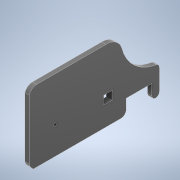
# Autodesk Inventor part: right_panel
Saved by Autodesk Inventor 2022 (Build 260153000, 153)
## iProperties
Created: 2021-06-17
Part Number: right_panel
Material: Plastic, Opaque Black
Document SubType Name: Modeling
Designer: kevin
Density: 0.952 g/cm^3
Appearance: Smooth - Black
Author: kevin
Autodesk Inventor part; units mm, degrees
ref_plane "YZ Plane" through (0, 0, 0) normal (1, 0, 0) x (0, 1, 0)
ref_plane "XZ Plane" through (0, 0, 0) normal (0, 1, 0) x (-1, 0, 0)
ref_plane "XY Plane" through (0, 0, 0) normal (0, 0, 1) x (1, 0, 0)
sketch "outline" plane through (0, 0, 0) normal (1, 0, 0) x (0, 1, 0)
  line L0 (0, 88.9038) -> (127, 88.9038) construction
  line L1 (127, 88.9038) -> (127, -88.8962) construction
  line L2 (127, -88.8962) -> (0, -88.8962) construction
  line L3 (0, -88.8962) -> (0, 88.9038) construction
  line L4 (0, 88.9038) -> (127, -88.8962) construction
  line L5 (127, 88.9038) -> (0, -88.8962) construction
  line L6 (-6.35, -82.5462) -> (38.1, -82.5462)
  line L7 (38.1, -82.5462) -> (38.1, -44.4462)
  line L8 (38.1, -44.4462) -> (-6.35, -44.4462)
  line L9 (-6.35, -44.4462) -> (-6.35, -82.5462)
  line L10 (4.9871, -50.7075) -> (22.0805, -50.7075) construction
  line L11 (22.0805, -50.7075) -> (22.0805, -80.6209) construction
  line L12 (22.0805, -80.6209) -> (4.9871, -80.6209) construction
  line L13 (4.9871, -80.6209) -> (4.9871, -50.7075) construction
  line L14 (179.262, 0.0038) -> (-38.2255, 0.0038) construction
  line L15 (0, 150.8125) -> (0, -173.0375) construction
  point P0 (63.5, 0.0038)
  point P1 (63.5, 0.0038)
  dimension "d0" = 177.8
  dimension "d1" = 127
  dimension "d2" = 38.1
  dimension "d3" = 44.45
  dimension "d4" = 6.35
  dimension "d5" = 6.35
  constraints: 24 end point, 4 horizontal, 4 parallel, 3 midpoint, 2 perpendicular, 2 vertical, 1 collinear, 1 point on line, 2 other
  measures "d0" distance of L0.end L1.end
  measures "d1" distance of L1.end L2.end
  measures "d2" distance of L8.end L6.start
  measures "d3" distance of L6.start L6.end
  measures "d4" distance between parallel lines of L6 L2
  measures "d5" distance between parallel lines of L9 L15
sketch "Sketch2" plane through (0, 0, 0) normal (1, 0, 0) x (0, 1, 0)
  line L0 (16.1492, -36.7509) -> (16.1492, 92.075)
  line L1 (25.5684, 98.5943) -> (113.7408, 98.5943)
  line L2 (121.8722, 87.4339) -> (121.8722, -14.7243)
  line L3 (38.1007, -44.45) -> (38.1007, -82.55)
  line L4 (38.1007, -44.45) -> (12.7007, -44.45)
  line L5 (38.1007, -82.55) -> (17.4632, -82.55)
  arc A0 (121.8722, 87.4339) -> (113.7408, 98.5943) centre (110.1475, 87.4339) ccw
  line L6 (31.7507, -44.45) -> (31.7507, 88.9) construction
  line L7 (25.4007, -44.45) -> (25.4007, 88.9) construction
  circle A1 centre (56.4395, 60.4012) radius 2.3813
  line L8 (0, -88.9) -> (117.475, -88.9) construction
  arc A2 (22.225, -82.55) -> (22.225, -93.6625) centre (22.225, -88.1063) ccw
  line L9 (22.225, -93.6625) -> (52.3875, -93.6625)
  arc A3 (104.2778, -38.5424) -> (58.7375, -88.9) centre (120.3654, -98.8617) ccw
  arc A4 (104.2778, -38.5424) -> (121.8722, -14.7243) centre (98.1639, -15.6185) ccw
  arc A5 (16.1492, -36.7509) -> (25.4007, -44.45) centre (23.7736, -36.9971) ccw
  arc A6 (25.5684, 98.5943) -> (16.1492, 92.075) centre (28.7116, 83.9887) ccw
  arc A7 (52.3875, -93.6625) -> (58.7375, -88.9) centre (53.0922, -87.9875) ccw
  point P0 (0, 0)
  point P1 (22.1466, -44.45)
  dimension "d6" = 6.35
  dimension "d7" = 6.35
  dimension "d8" = 4.7625
  dimension "d9" = 24.6888
  dimension "d10" = 149.3012
  constraints: 20 end point, 14 point on circle, 8 centre point, 8 horizontal, 6 vertical, 4 tangent, 2 midpoint, 2 point on line
  measures "d6" distance between parallel lines of L6 L3
  measures "d7" distance between parallel lines of L7 L6
  measures "d8" diameter of A1
  measures "d9" distance from line of L6 A1.centre
  measures "d10" distance from line of A1.centre L8
extrude "main right panel" add sketch "Sketch2" along normal blind 6.35 contours L0 A6 L1 A0 L2 A4 A3 A7 L9 A2 L5 L3 L4 A5
sketch "rat icon raw" plane through (6.35, 0, 0) normal (1, 0, 0) x (0, 0, -1)
  line L0 (-53.1267, 106.3625) -> (-10.9673, 106.3625) construction
  line L1 (-10.9673, 106.3625) -> (-10.9673, 68.2625) construction
  line L2 (-10.9673, 68.2625) -> (-53.1267, 68.2625) construction
  line L3 (-53.1267, 68.2625) -> (-53.1267, 106.3625) construction
  line L4 (-80.9625, 106.3625) -> (-14.2875, 106.3625) construction
  line L5 (-80.9625, 68.2625) -> (-14.2875, 68.2625) construction
  point P0 (0, 0)
  constraints: 4 end point, 4 horizontal, 2 collinear, 2 other
sketch "Sketch6" plane through (6.35, 0, 0) normal (1, 0, 0) x (0, 0, -1)
  line L0 (-90.482, 107.6466) -> (-76.2, 109.283)
  line L1 (-76.2, 109.283) -> (-77.7875, 104.5205)
  line L2 (-77.7875, 104.5205) -> (-82.9028, 104.5205)
  line L3 (-82.9028, 104.5205) -> (-81.9686, 96.3676)
  line L4 (-81.9686, 96.3676) -> (-86.8566, 96.3676)
  line L5 (-86.8566, 96.3676) -> (-85.1932, 104.5205)
  line L6 (-85.1932, 104.5205) -> (-91.0958, 104.5205)
  line L7 (-91.0958, 104.5205) -> (-90.482, 107.6466)
  line L8 (-73.7939, 108.2258) -> (-76.2, 96.3676)
  line L9 (-76.2, 96.3676) -> (-73.7454, 96.3676)
  line L10 (-73.7454, 96.3676) -> (-73.0058, 100.0125)
  line L11 (-73.0058, 100.0125) -> (-71.4375, 99.6943)
  line L12 (-71.4375, 99.6943) -> (-71.4375, 96.3676)
  line L13 (-71.4375, 96.3676) -> (-69.85, 96.3676)
  line L14 (-69.85, 96.3676) -> (-69.85, 101.3768)
  line L15 (-69.85, 101.3768) -> (-72.5181, 102.4162)
  line L16 (-72.5181, 102.4162) -> (-72.5181, 108.2258)
  line L17 (-72.5181, 108.2258) -> (-73.7939, 108.2258)
  line L18 (-65.1277, 100.0518) -> (-60.3603, 100.4265)
  line L19 (-60.3603, 100.4265) -> (-61.915, 103.1887)
  line L20 (-61.915, 103.1887) -> (-65.8535, 103.1887)
  line L21 (-65.8535, 103.1887) -> (-67.3493, 100.0125)
  line L22 (-67.3493, 100.0125) -> (-65.851, 96.3676)
  line L23 (-65.851, 96.3676) -> (-61.9125, 96.3676)
  line L24 (-61.9125, 96.3676) -> (-61.0199, 98.263)
  line L25 (-61.0199, 98.263) -> (-64.9627, 97.9531)
  line L26 (-64.9627, 97.9531) -> (-65.1277, 100.0518)
  line L27 (-92.0732, 92.0678) -> (-88.8982, 71.4303)
  line L28 (-88.8982, 71.4303) -> (-84.5851, 71.4303)
  line L29 (-84.5851, 71.4303) -> (-88.1511, 81.4759)
  line L30 (-88.1511, 81.4759) -> (-79.1594, 71.8603)
  line L31 (-79.1594, 71.8603) -> (-76.0148, 73.6303)
  line L32 (-76.0148, 73.6303) -> (-85.6976, 83.1021)
  line L33 (-85.6976, 83.1021) -> (-79.375, 84.8156)
  line L34 (-79.375, 84.8156) -> (-80.2421, 90.4519)
  line L35 (-80.2421, 90.4519) -> (-86.7416, 93.5127)
  line L36 (-86.7416, 93.5127) -> (-92.0732, 92.0678)
  line L37 (-88.9716, 89.5226) -> (-87.785, 85.1441)
  line L38 (-87.785, 85.1441) -> (-83.4928, 86.9084)
  line L39 (-83.4928, 86.9084) -> (-85.2835, 90.09)
  line L40 (-85.2835, 90.09) -> (-88.9716, 89.5226)
  line L41 (-64.6954, 101.9367) -> (-64.9301, 100.9638)
  line L42 (-64.9301, 100.9638) -> (-62.5497, 101.2457)
  line L43 (-62.5497, 101.2457) -> (-63.5298, 102.4036)
  line L44 (-63.5298, 102.4036) -> (-64.6954, 101.9367)
  line L45 (-76.7521, 84.3599) -> (-74.2642, 86.4657)
  line L46 (-74.2642, 86.4657) -> (-67.2415, 87.5488)
  line L47 (-67.2415, 87.5488) -> (-63.3352, 73.4152)
  line L48 (-63.3352, 73.4152) -> (-66.1281, 72.9844)
  line L49 (-66.1281, 72.9844) -> (-66.4584, 75.1263)
  line L50 (-66.4584, 75.1263) -> (-68.2934, 73.264)
  line L51 (-68.2934, 73.264) -> (-73.1451, 72.5157)
  line L52 (-73.1451, 72.5157) -> (-74.9114, 74.256)
  line L53 (-74.9114, 74.256) -> (-75.6403, 78.9817)
  line L54 (-75.6403, 78.9817) -> (-74.0283, 80.6177)
  line L55 (-74.0283, 80.6177) -> (-67.6783, 81.5971)
  line L56 (-67.6783, 81.5971) -> (-69.2347, 85.4828)
  line L57 (-69.2347, 85.4828) -> (-73.6131, 84.2727)
  line L58 (-73.6131, 84.2727) -> (-74.9869, 83.1098)
  line L59 (-74.9869, 83.1098) -> (-76.7521, 84.3599)
  line L60 (-72.0695, 78.6877) -> (-72.3134, 78.5673)
  line L61 (-72.3134, 78.5673) -> (-72.3134, 75.1263)
  line L62 (-72.3134, 75.1263) -> (-68.8702, 75.1263)
  line L63 (-68.8702, 75.1263) -> (-67.1347, 76.6189)
  line L64 (-67.1347, 76.6189) -> (-68.5083, 79.4017)
  line L65 (-68.5083, 79.4017) -> (-72.0695, 78.6877)
  line L66 (-61.8214, 93.0066) -> (-61.1645, 86.6956)
  line L67 (-61.1645, 86.6956) -> (-63.0921, 86.495)
  line L68 (-63.0921, 86.495) -> (-63.0921, 83.125)
  line L69 (-63.0921, 83.125) -> (-60.7929, 83.125)
  line L70 (-60.7929, 83.125) -> (-60.1157, 76.6189)
  line L71 (-60.1157, 76.6189) -> (-57.8831, 74.256)
  line L72 (-57.8831, 74.256) -> (-52.8496, 74.78)
  line L73 (-52.8496, 74.78) -> (-53.882, 75.8726)
  line L74 (-53.882, 75.8726) -> (-57.8951, 76.85)
  line L75 (-57.8951, 76.85) -> (-58.5482, 83.125)
  line L76 (-58.5482, 83.125) -> (-55.3914, 82.3562)
  line L77 (-55.3914, 82.3562) -> (-56.9753, 85.3316)
  line L78 (-56.9753, 85.3316) -> (-58.9439, 86.9267)
  line L79 (-59.6008, 93.2377) -> (-61.8214, 93.0066)
  line L80 (-59.6008, 93.2377) -> (-58.9439, 86.9267)
  line L81 (-90.3273, 66.9011) -> (-92.3025, 43.7452)
  line L82 (-92.3025, 43.7452) -> (-83.6552, 43.0076)
  line L83 (-83.6552, 43.0076) -> (-80.3451, 45.7207)
  line L84 (-80.3451, 45.7207) -> (-80.3451, 53.0314)
  line L85 (-80.3451, 53.0314) -> (-82.9028, 54.9333)
  line L86 (-82.9028, 54.9333) -> (-87.9789, 56.2066)
  line L87 (-87.9789, 56.2066) -> (-85.4408, 67.3056)
  line L88 (-85.4408, 67.3056) -> (-90.3273, 66.9011)
  line L89 (-89.0531, 51.5088) -> (-89.0531, 47.7554)
  line L90 (-89.0531, 47.7554) -> (-85.6389, 46.9746)
  line L91 (-85.6389, 46.9746) -> (-83.6628, 49.6321)
  line L92 (-83.6628, 49.6321) -> (-84.778, 53.0314)
  line L93 (-84.778, 53.0314) -> (-89.0531, 51.6289)
  line L94 (-77.7875, 66.9369) -> (-80.6353, 64.5461)
  line L95 (-80.6353, 64.5461) -> (-79.5703, 56.8049)
  line L96 (-79.5703, 56.8049) -> (-75.7895, 55.9249)
  line L97 (-75.7895, 55.9249) -> (-71.5386, 59.4937)
  line L98 (-71.5386, 59.4937) -> (-72.3897, 65.6805)
  line L99 (-72.3897, 65.6805) -> (-77.7875, 66.9369)
  line L100 (-77.7875, 62.5871) -> (-77.7875, 58.634)
  line L101 (-77.7875, 58.634) -> (-75.0886, 58.634)
  line L102 (-75.0886, 58.634) -> (-74.7055, 63.4204)
  line L103 (-74.7055, 63.4204) -> (-76.6131, 63.573)
  line L104 (-76.6131, 63.573) -> (-77.7875, 62.5871)
  line L105 (-68.4972, 70.5753) -> (-68.5693, 68.2366)
  line L106 (-68.5693, 68.2366) -> (-66.2151, 58.3858)
  line L107 (-66.2151, 58.3858) -> (-72.6469, 52.0948)
  line L108 (-72.6469, 52.0948) -> (-70.8707, 49.9791)
  line L109 (-70.8707, 49.9791) -> (-54.5671, 67.2736)
  line L110 (-54.5671, 67.2736) -> (-57.5505, 65.6195)
  line L111 (-57.5505, 65.6195) -> (-64.4697, 61.7832)
  line L112 (-64.4697, 61.7832) -> (-66.675, 71.0108)
  line L113 (-66.675, 71.0108) -> (-68.4972, 70.5753)
  line L114 (-43.6156, 68.0273) -> (-44.641, 70.5217)
  line L115 (-44.641, 70.5217) -> (-52.7086, 70.5217)
  line L116 (-52.7086, 70.5217) -> (-52.7086, 65.9787)
  line L117 (-52.7086, 65.9787) -> (-47.0988, 58.9781)
  line L118 (-47.0988, 58.9781) -> (-52.7086, 57.21)
  line L119 (-52.7086, 57.21) -> (-52.0224, 55.0327)
  line L120 (-52.0224, 55.0327) -> (-43.2547, 56.1214)
  line L121 (-43.2547, 56.1214) -> (-43.2547, 60.8776)
  line L122 (-43.2547, 60.8776) -> (-48.8355, 67.3792)
  line L123 (-48.8355, 67.3792) -> (-43.6156, 68.0273)
  point P0 (0, 0)
  constraints: 248 end point, 33 perpendicular, 23 parallel, 17 point on line, 6 vertical, 4 horizontal
extrude "the rat boys words" [suppressed]
sketch "detail lines" plane through (6.35, 0, 0) normal (1, 0, 0) x (0, 0, -1)
  line L0 (41.275, 68.2625) -> (-1.5875, 68.2625)
  line L1 (-1.5875, 68.2625) -> (-1.5875, 107.95)
  arc A0 (41.275, 68.2625) -> (-1.5875, 107.95) centre (-4.3356, 61.9925) ccw
  line L2 (-4.1415, 110.938) -> (-4.1415, 28.575)
  line L3 (-4.1415, 28.575) -> (31.75, 28.575)
  arc A1 (44.45, 66.675) -> (-4.1415, 110.938) centre (-10.0865, 55.6085) ccw
  line L4 (44.45, 66.675) -> (44.45, 41.275)
  arc A2 (44.45, 41.275) -> (31.75, 28.575) centre (44.45, 28.575) ccw
  line L5 (-1.5875, 61.9925) -> (4.7625, 61.9925) construction
  line L6 (-1.5875, 60.4851) -> (4.7625, 60.4851)
  line L7 (4.7625, 63.5) -> (-1.5875, 63.5)
  arc A3 (-1.5875, 63.5) -> (-1.5875, 60.4851) centre (-1.5875, 61.9925) ccw
  arc A4 (4.7625, 60.4851) -> (4.7625, 63.5) centre (4.7625, 61.9925) ccw
  line L8 (35.4697, 23.6503) -> (-87.3125, 23.6503)
  line L9 (-87.4339, 115.8875) -> (19.8438, 115.8875)
  arc A5 (33.3375, 107.95) -> (19.8438, 115.8875) centre (17.1097, 95.8012) ccw
  line L10 (-87.4339, 115.8875) -> (-87.4339, 114.3)
  line L11 (-87.4339, 114.3) -> (18.8487, 114.3)
  arc A6 (31.75, 107.1391) -> (18.8487, 114.3) centre (18.8487, 99.0979) ccw
  line L12 (31.75, 107.1391) -> (33.3375, 107.95)
  line L13 (-87.3125, 23.6503) -> (-87.3125, 21.5255)
  line L14 (-87.3125, 21.5255) -> (35.4697, 21.5255)
  line L15 (35.4697, 21.5255) -> (35.4697, 23.6503)
  point P0 (0, 0)
  point P1 (1.5875, 61.9925)
  constraints: 34 end point, 14 point on circle, 7 centre point, 5 perpendicular, 5 tangent, 4 horizontal, 4 vertical, 1 midpoint, 1 parallel
extrude "car details extrusion" add sketch "detail lines" along normal blind 2.54
sketch "rat sketch" plane through (6.35, 0, 0) normal (1, 0, 0) x (0, 0, -1)
  spline S0 degree 4 poles (-25.1113, 40.168) (-30.3286, 62.8002) (-40.2895, 47.0939) (-91.8199, 45.4722) (-69.0311, 66.7314) knots 0 0 0 0 0 1 1 1 1 1
  spline S1 degree 4 poles (-25.1113, 40.168) (-44.8827, 65.0652) (-62.3129, 21.5895) (-100.0449, 58.8688) (-70.6074, 74.0707) knots 0 0 0 0 0 1 1 1 1 1
  arc A0 (-69.0311, 66.7314) -> (-67.585, 61.8172) centre (-67.0769, 64.6366) ccw
  arc A1 (-49.2116, 58.7947) -> (-67.585, 61.8172) centre (-65.5506, 16.8269) ccw
  line L0 (-49.2116, 58.7947) -> (-50.6913, 60.6928)
  line L1 (-50.6913, 60.6928) -> (-46.1556, 58.7947)
  line L2 (-46.1556, 58.7947) -> (-48.7906, 62.1746)
  line L3 (-48.7906, 62.1746) -> (-44.7522, 60.4847)
  line L4 (-44.7522, 60.4847) -> (-47.0983, 63.4939)
  arc A2 (-55.3235, 64.9029) -> (-47.0983, 63.4939) centre (-49.5283, 74.0213) ccw
  arc A3 (-55.3235, 64.9029) -> (-61.4396, 83.2385) centre (-66.0407, 71.5159) ccw
  arc A4 (-55.3235, 64.9029) -> (-61.4396, 83.2385) centre (-62.9686, 72.5406) ccw
  arc A5 (-54.0945, 66.3736) -> (-40.9879, 66.7314) centre (-47.8743, 78.7553) ccw
  arc A6 (-40.9879, 66.7314) -> (-36.1311, 63.3712) centre (-37.5728, 66.4775) ccw
  arc A7 (-33.4791, 95.4623) -> (-76.7213, 69.5945) centre (-48.4257, 71.3709) ccw
  arc A8 (-36.1311, 63.3712) -> (-34.9888, 58.791) centre (16.1312, 73.9736) ccw
  line L5 (-34.9888, 58.791) -> (-34.9888, 62.1708)
  line L6 (-34.9888, 62.1708) -> (-32.1742, 61.0684)
  line L7 (-32.1742, 61.0684) -> (-30.8802, 58.791)
  line L8 (-30.8802, 58.791) -> (-31.2041, 61.6196)
  line L9 (-31.2041, 61.6196) -> (-32.1742, 62.8915)
  line L10 (-32.1742, 62.8915) -> (-30.6857, 62.8915)
  line L11 (-30.6857, 62.8915) -> (-29.0402, 60.4346)
  line L12 (-29.0402, 60.4346) -> (-29.0402, 62.3815)
  line L13 (-29.0402, 62.3815) -> (-29.9306, 63.7109)
  line L14 (-29.9306, 63.7109) -> (-27.2529, 62.8915)
  line L15 (-27.2529, 62.8915) -> (-28.2579, 64.392)
  arc A9 (-28.2579, 64.392) -> (-33.7777, 64.8449) centre (-31.6378, 57.0631) ccw
  arc A10 (-34.8841, 70.1283) -> (-33.7777, 64.8449) centre (-32.3651, 67.8983) ccw
  arc A11 (-34.8841, 70.1283) -> (-23.8004, 78.7218) centre (-46.3737, 96.3917) ccw
  arc A12 (-23.8004, 78.7218) -> (-15.5306, 77.1344) centre (-17.1285, 91.1448) ccw
  line L16 (-15.5306, 77.1344) -> (-13.4262, 78.7736)
  arc A13 (-13.4262, 78.7736) -> (-12.5498, 83.2524) centre (-12.73, 80.9625) ccw
  line L17 (-12.5498, 83.2524) -> (-17.1338, 91.6691)
  line L18 (-17.1338, 91.6691) -> (-22.5552, 93.9422)
  arc A14 (-24.7828, 98.5157) -> (-22.5552, 93.9422) centre (-22.0776, 97.0041) ccw
  arc A15 (-24.7828, 98.5157) -> (-27.2583, 102.3227) centre (-27.0229, 99.7674) ccw
  arc A16 (-30.6895, 96.6707) -> (-27.2583, 102.3227) centre (-32.5957, 101.6955) ccw
  arc A17 (-30.6895, 96.6707) -> (-33.4791, 95.4623) centre (-19.0133, 65.8926) ccw
  arc A18 (-17.8515, 86.2944) -> (-24.7683, 89.3504) centre (-22.6941, 84.6895) ccw
  arc A19 (-24.7558, 89.356) -> (-17.8515, 86.2944) centre (-19.1737, 92.6286) ccw
  arc A20 (-32.5957, 93.9422) -> (-29.4854, 87.2366) centre (-28.196, 91.9088) ccw
  arc A21 (-25.7638, 91.6691) -> (-32.5957, 93.9422) centre (-30.7455, 88.0996) ccw
  arc A22 (-26.408, 91.1448) -> (-31.0346, 92.4063) centre (-29.6597, 88.3339) ccw
  arc A23 (-31.0346, 92.4063) -> (-29.0402, 87.4607) centre (-25.1113, 91.9201) ccw
  line L19 (-29.0402, 87.4607) -> (-29.4854, 87.2366)
  line L20 (-26.408, 91.1448) -> (-25.7638, 91.6691)
  line L21 (-19.1737, 77.1927) -> (-22.6941, 72.5406)
  line L22 (-22.6941, 72.5406) -> (-22.6941, 71.6578)
  line L23 (-22.6941, 71.6578) -> (-18.6565, 77.1266)
  line L24 (-20.5712, 69.8924) -> (-17.5596, 76.9468)
  line L25 (-20.5712, 69.8924) -> (-20.5712, 70.2775)
  line L26 (-20.5712, 70.2775) -> (-17.8411, 77.0616)
  line L27 (-17.5935, 76.8675) -> (-18.3698, 71.0148)
  line L28 (-18.3698, 71.0148) -> (-18.1898, 70.2775)
  line L29 (-18.1898, 70.2775) -> (-17.2434, 76.8211)
  line L30 (-17.2434, 76.8211) -> (-17.2434, 77.0441)
  line L31 (-12.5498, 83.2524) -> (-9.4887, 86.2944)
  line L32 (-9.4887, 86.2944) -> (-11.9194, 84.6895)
  line L33 (-11.9194, 84.6895) -> (-6.9637, 91.1448)
  line L34 (-6.9637, 91.1448) -> (-12.5498, 85.492)
  line L35 (-12.5498, 85.492) -> (-11.3289, 88.6625)
  line L36 (-11.3289, 88.6625) -> (-13.0786, 85.5794)
  line L37 (-13.0786, 85.5794) -> (-13.5578, 85.1032)
  point P0 (0, 0)
  point P1 (-32.5957, 51.1893)
  point P2 (-50.6956, 51.4518)
  point P3 (-71.9355, 54.0894)
  point P4 (-46.3737, 47.5886)
  point P5 (-67.5516, 46.5674)
  point P6 (-79.7754, 55.7354)
  point P7 (-18.6565, 77.1266)
  constraints: 76 end point, 56 point on circle, 24 centre point, 6 parallel, 5 vertical, 3 point on line, 2 tangent, 1 coincident, 1 horizontal, 1 perpendicular, 14 other
extrude "rat extrusion" [suppressed]
mirror "Mirror1" about plane through (0, 0, 0) normal (1, 0, 0) remove original yes
sketch "Sketch7" plane through (-6.35, 25.5684, 98.5943) normal (-1, 0, 0) x (0, 0, 1)
  line L0 (-83.8164, 82.6102) -> (-17.4625, 82.6102) construction
  line L1 (-17.4625, 82.6102) -> (-17.4625, 36.5125) construction
  line L2 (-17.4625, 36.5125) -> (-83.8164, 36.5125) construction
  line L3 (-83.8164, 36.5125) -> (-83.8164, 82.6102) construction
  line L4 (-82.8534, 82.6102) -> (-79.4482, 82.6102)
  spline S0 degree 2 poles (-79.4482, 82.6102) (-76.043, 82.6102) (-73.6287, 82.0799) (-72.1075, 79.9168) (-72.1075, 77.5583) knots 0 0 0 1 2 3 3 3
  spline S1 degree 2 poles (-72.1075, 77.5583) (-72.1075, 75.3951) (-73.1821, 73.9018) (-74.7591, 73.7483) knots 0 0 0 1 2 2 2
  spline S2 degree 2 poles (-74.7591, 73.7483) (-73.3356, 73.3994) (-72.3447, 72.2132) (-72.1075, 71.2223) (-72.1075, 68.9755) knots 0 0 0 1 2 3 3 3
  line L5 (-72.1075, 68.9755) -> (-72.1075, 64.0909)
  line L6 (-72.1075, 64.0909) -> (-76.5873, 64.0909)
  line L7 (-76.5873, 64.0909) -> (-76.5873, 70.2454)
  spline S3 degree 2 poles (-76.5873, 70.2454) (-76.5873, 71.7247) (-77.0478, 72.4365) (-78.0387, 72.4365) knots 0 0 0 1 2 2 2
  line L8 (-78.0387, 72.4365) -> (-78.0387, 64.0909)
  line L9 (-78.0387, 64.0909) -> (-82.8534, 64.0909)
  line L10 (-82.8534, 64.0909) -> (-82.8534, 82.6102)
  line L11 (-78.0387, 79.4423) -> (-78.0387, 75.3253)
  spline S4 degree 2 poles (-78.0387, 75.3253) (-77.2293, 75.3253) (-76.5873, 75.7719) (-76.5873, 77) knots 0 0 0 1 2 2 2
  line L12 (-76.5873, 77) -> (-76.5873, 78.0188)
  spline S5 degree 2 poles (-76.5873, 78.0188) (-76.5873, 78.898) (-77.2153, 79.4423) (-78.0387, 79.4423) knots 0 0 0 1 2 2 2
  line L13 (-61.9198, 82.6102) -> (-59.1565, 64.0909)
  line L14 (-59.1565, 64.0909) -> (-64.0969, 64.0909)
  line L15 (-64.0969, 64.0909) -> (-64.3481, 67.4264)
  line L16 (-64.3481, 67.4264) -> (-66.0646, 67.4264)
  line L17 (-66.0646, 67.4264) -> (-66.3438, 64.0909)
  line L18 (-66.3438, 64.0909) -> (-71.3399, 64.0909)
  line L19 (-71.3399, 64.0909) -> (-68.8977, 82.6102)
  line L20 (-68.8977, 82.6102) -> (-61.9198, 82.6102)
  spline S6 degree 2 poles (-64.4737, 70.706) (-64.8226, 73.846) (-65.1994, 78.4793) knots 0 0 0 1 1 1
  spline S7 degree 2 poles (-65.1994, 78.4793) (-65.9251, 73.1622) (-66.1205, 70.706) knots 0 0 0 1 1 1
  line L21 (-66.1205, 70.706) -> (-64.4737, 70.706)
  line L22 (-48.6339, 82.6102) -> (-48.6339, 78.898)
  line L23 (-48.6339, 78.898) -> (-51.4948, 78.898)
  line L24 (-51.4948, 78.898) -> (-51.4948, 64.0909)
  line L25 (-51.4948, 64.0909) -> (-56.3096, 64.0909)
  line L26 (-56.3096, 64.0909) -> (-56.3096, 78.898)
  line L27 (-56.3096, 78.898) -> (-59.1565, 78.898)
  line L28 (-59.1565, 78.898) -> (-59.1565, 82.6102)
  line L29 (-59.1565, 82.6102) -> (-48.6339, 82.6102)
  line L30 (-70.4607, 59.7502) -> (-65.6599, 59.7502)
  spline S8 degree 2 poles (-65.6599, 59.7502) (-63.3712, 59.7502) (-61.0266, 59.0385) (-59.5892, 56.8754) (-59.5892, 54.475) knots 0 0 0 1 2 3 3 3
  spline S9 degree 2 poles (-59.5892, 54.475) (-59.5892, 52.8561) (-60.6079, 51.5722) (-62.1152, 51.2372) knots 0 0 0 1 2 2 2
  spline S10 degree 2 poles (-62.1152, 51.2372) (-60.4405, 50.8465) (-59.2542, 49.102) (-59.2542, 47.2877) knots 0 0 0 1 2 2 2
  line L31 (-59.2542, 47.2877) -> (-59.2542, 45.5851)
  spline S11 degree 2 poles (-59.2542, 45.5851) (-59.2542, 43.7011) (-60.1055, 41.9008) (-61.9896, 41.2309) (-64.8924, 41.2309) knots 0 0 0 1 2 3 3 3
  line L32 (-64.8924, 41.2309) -> (-70.4607, 41.2309)
  line L33 (-70.4607, 41.2309) -> (-70.4607, 59.7502)
  line L34 (-65.646, 49.5765) -> (-65.646, 44.3989)
  spline S12 degree 2 poles (-65.646, 44.3989) (-64.6272, 44.4268) (-64.069, 44.999) (-64.069, 46.1294) knots 0 0 0 1 2 2 2
  line L35 (-64.069, 46.1294) -> (-64.069, 47.846)
  spline S13 degree 2 poles (-64.069, 47.846) (-64.069, 49.0462) (-64.5714, 49.5486) (-65.646, 49.5765) knots 0 0 0 1 2 2 2
  line L36 (-65.646, 56.5823) -> (-65.646, 52.4653)
  spline S14 degree 2 poles (-65.646, 52.4653) (-65.3389, 52.4793) (-65.1715, 52.4793) knots 0 0 0 1 1 1
  spline S15 degree 2 poles (-65.1715, 52.4793) (-64.4597, 52.4793) (-64.069, 53.1771) (-64.069, 54.8239) knots 0 0 0 1 2 2 2
  spline S16 degree 2 poles (-64.069, 54.8239) (-64.069, 55.6891) (-64.3899, 56.3869) (-64.9063, 56.5683) (-65.646, 56.5823) knots 0 0 0 1 2 3 3 3
  spline S17 degree 2 poles (-46.5266, 48.9066) (-46.5266, 46.1155) (-46.7917, 43.7988) (-48.1733, 41.8729) (-50.5319, 40.8402) (-52.0949, 40.8402) knots 0 0 0 1 2 3 4 4 4
  spline S18 degree 2 poles (-52.0949, 40.8402) (-53.5882, 40.8402) (-55.9467, 41.8171) (-57.3842, 43.7569) (-57.6633, 46.0457) (-57.6633, 48.9066) knots 0 0 0 1 2 3 4 4 4
  line L37 (-57.6633, 48.9066) -> (-57.6633, 52.0746)
  spline S19 degree 2 poles (-57.6633, 52.0746) (-57.6633, 54.8657) (-57.3981, 57.1824) (-56.0165, 59.1083) (-53.658, 60.141) (-52.0949, 60.141) knots 0 0 0 1 2 3 4 4 4
  spline S20 degree 2 poles (-52.0949, 60.141) (-50.6016, 60.141) (-48.2431, 59.1641) (-46.8057, 57.2242) (-46.5266, 54.9355) (-46.5266, 52.0746) knots 0 0 0 1 2 3 4 4 4
  line L38 (-46.5266, 52.0746) -> (-46.5266, 48.9066)
  spline S21 degree 2 poles (-51.3413, 54.9913) (-51.3413, 56.2753) (-51.6204, 57.001) (-52.067, 57.001) knots 0 0 0 1 2 2 2
  spline S22 degree 2 poles (-52.067, 57.001) (-52.4438, 57.001) (-52.8485, 56.4148) (-52.8485, 54.9913) knots 0 0 0 1 2 2 2
  line L39 (-52.8485, 54.9913) -> (-52.8485, 46.3527)
  spline S23 degree 2 poles (-52.8485, 46.3527) (-52.8485, 44.7338) (-52.5834, 43.9802) (-52.1089, 43.9802) knots 0 0 0 1 2 2 2
  spline S24 degree 2 poles (-52.1089, 43.9802) (-51.6204, 43.9802) (-51.3413, 44.8455) (-51.3413, 46.4783) knots 0 0 0 1 2 2 2
  line L40 (-51.3413, 46.4783) -> (-51.3413, 54.9913)
  line L41 (-34.4548, 59.7502) -> (-37.9717, 47.9297)
  line L42 (-37.9717, 47.9297) -> (-37.9717, 41.2309)
  line L43 (-37.9717, 41.2309) -> (-42.4375, 41.2309)
  line L44 (-42.4375, 41.2309) -> (-42.4375, 47.9297)
  line L45 (-42.4375, 47.9297) -> (-45.8288, 59.7502)
  line L46 (-45.8288, 59.7502) -> (-41.4048, 59.7502)
  spline S25 degree 2 poles (-41.4048, 59.7502) (-40.3721, 54.3214) (-40.2325, 52.4514) knots 0 0 0 1 1 1
  spline S26 degree 2 poles (-40.2325, 52.4514) (-39.8138, 55.41) (-38.8788, 59.7502) knots 0 0 0 1 1 1
  line L47 (-38.8788, 59.7502) -> (-34.4548, 59.7502)
  line L48 (-23.4437, 54.154) -> (-27.9235, 54.154)
  line L49 (-27.9235, 54.154) -> (-27.9235, 55.5216)
  spline S27 degree 2 poles (-27.9235, 55.5216) (-27.9235, 56.4706) (-28.2585, 57.001) (-28.6632, 57.001) knots 0 0 0 1 2 2 2
  spline S28 degree 2 poles (-28.6632, 57.001) (-29.0958, 57.001) (-29.5424, 56.2892) (-29.5424, 55.5775) knots 0 0 0 1 2 2 2
  spline S29 degree 2 poles (-29.5424, 55.5775) (-29.5424, 54.6564) (-29.2912, 54.1819) knots 0 0 0 1 1 1
  spline S30 degree 2 poles (-29.2912, 54.1819) (-29.04, 53.7074) (-27.9235, 53.0515) knots 0 0 0 1 1 1
  spline S31 degree 2 poles (-27.9235, 53.0515) (-24.7137, 51.1395) (-23.8763, 49.9114) knots 0 0 0 1 1 1
  spline S32 degree 2 poles (-23.8763, 49.9114) (-23.039, 48.6833) (-23.039, 45.9619) knots 0 0 0 1 1 1
  spline S33 degree 2 poles (-23.039, 45.9619) (-23.039, 43.9802) (-23.9601, 42.1101) (-26.6256, 40.8402) (-28.3841, 40.8402) knots 0 0 0 1 2 3 3 3
  spline S34 degree 2 poles (-28.3841, 40.8402) (-30.31, 40.8402) (-33.0453, 42.3055) (-33.8966, 44.5664) (-33.8966, 46.6458) knots 0 0 0 1 2 3 3 3
  line L50 (-33.8966, 46.6458) -> (-33.8966, 47.8599)
  line L51 (-33.8966, 47.8599) -> (-29.4168, 47.8599)
  line L52 (-29.4168, 47.8599) -> (-29.4168, 45.613)
  spline S35 degree 2 poles (-29.4168, 45.613) (-29.4168, 44.5803) (-29.04, 43.9802) (-28.5655, 43.9802) knots 0 0 0 1 2 2 2
  spline S36 degree 2 poles (-28.5655, 43.9802) (-28.077, 43.9802) (-27.6165, 44.7338) (-27.6165, 45.4735) knots 0 0 0 1 2 2 2
  spline S37 degree 2 poles (-27.6165, 45.4735) (-27.6165, 47.1063) (-28.0631, 47.6087) knots 0 0 0 1 1 1
  spline S38 degree 2 poles (-28.0631, 47.6087) (-28.5236, 48.1111) (-30.3239, 49.2974) knots 0 0 0 1 1 1
  spline S39 degree 2 poles (-30.3239, 49.2974) (-32.1103, 50.4836) (-33.2825, 51.5582) (-34.0501, 53.4562) (-34.0501, 54.9355) knots 0 0 0 1 2 3 3 3
  spline S40 degree 2 poles (-34.0501, 54.9355) (-34.0501, 57.0707) (-32.9616, 59.0385) (-30.5332, 60.141) (-28.8167, 60.141) knots 0 0 0 1 2 3 3 3
  spline S41 degree 2 poles (-28.8167, 60.141) (-26.9466, 60.141) (-24.295, 58.9269) (-23.4437, 57.0847) (-23.4437, 54.8797) knots 0 0 0 1 2 3 3 3
  line L53 (-23.4437, 54.8797) -> (-23.4437, 54.154)
  point P0 (-98.5943, -25.5684)
  constraints: 2 other
extrude "rat boys ketters" add sketch "Sketch7" along normal blind 6.35
sketch "Sketch8" plane through (0, 25.5684, 98.5943) normal (1, 0, 0) x (0, 0, -1)
  line L0 (143.0443, 12.5322) -> (122.7243, 12.5322) construction
  line L1 (122.7243, 12.5322) -> (122.7243, 20.1522) construction
  line L2 (122.7243, 20.1522) -> (110.0243, 20.1522)
  line L3 (110.0243, 20.1522) -> (110.0243, 32.8522)
  line L4 (110.0243, 32.8522) -> (122.7243, 32.8522)
  line L5 (122.7243, 32.8522) -> (122.7243, 20.1522)
  point P0 (98.5943, -25.5684)
  dimension "d52" = 20.32
  dimension "d53" = 7.62
  dimension "d54" = 12.7
  dimension "d55" = 12.7
  constraints: 12 end point, 2 horizontal, 2 parallel, 2 perpendicular
  measures "d52" distance of L0.start L0.end
  measures "d53" distance of L0.end L1.end
  measures "d54" distance of L4.end L1.end
  measures "d55" distance of L3.end L4.end
extrude "arduino plug hole" cut sketch "Sketch8" against normal blind 11.1125
body "Solid1"
